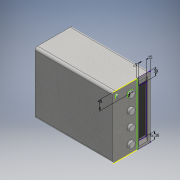
# Autodesk Inventor part: labortap1
Saved by Autodesk Inventor 2016 (Build 200138000, 138)
## iProperties
Created: 2017-12-27
Part Number: labortap1
Material: Generic
Document SubType Name: Modeling
Designer: Barna
Density: 1 g/cm^3
Appearance: Default
Author: Barna
Autodesk Inventor part; units mm, degrees
ref_plane "YZ Plane" through (0, 0, 0) normal (1, 0, 0) x (0, 1, 0)
ref_plane "XZ Plane" through (0, 0, 0) normal (0, 1, 0) x (-1, 0, 0)
ref_plane "XY Plane" through (0, 0, 0) normal (0, 0, 1) x (1, 0, 0)
sketch "Sketch1" plane through (0, 0, 0) normal (1, 0, 0) x (0, 1, 0)
  line L0 (0, 0) -> (155, 0)
  line L1 (155, 0) -> (155, -255)
  line L2 (155, -255) -> (0, -255)
  line L3 (0, -255) -> (0, 0)
  dimension "d1" = 255
  dimension "d2" = 155
  constraints: 8 end point, 2 parallel, 1 horizontal, 1 perpendicular
  measures "d1" distance of L0.end L1.end
  measures "d2" distance of L1.end L2.end
extrude "Extrusion1" add sketch "Sketch1" against normal blind 320
sketch "Sketch2" plane through (0, 0, 0) normal (1, 0, 0) x (0, 0, -1)
  line L0 (0, 0) -> (0, 155) projected
  line L1 (255, 155) -> (255, 0) projected
  line L2 (0, 155) -> (255, 155)
  line L3 (255, 155) -> (255, 99.4837)
  line L4 (255, 99.4837) -> (0, 99.4837)
  line L5 (0, 99.4837) -> (0, 155)
  line L6 (30, 140) -> (225, 140)
  line L7 (225, 140) -> (225, 104.4837)
  line L8 (225, 104.4837) -> (30, 104.4837)
  line L9 (30, 104.4837) -> (30, 140)
  dimension "d8" = 15
  dimension "d9" = 5
  dimension "d10" = 30
  dimension "d11" = 30
  constraints: 16 end point, 4 parallel, 2 horizontal, 2 perpendicular, 1 point on line
  measures "d8" distance between parallel lines of L6 L2
  measures "d9" distance between parallel lines of L4 L8
  measures "d10" distance between parallel lines of L0 L9
  measures "d11" distance between parallel lines of L1 L7
extrude "Extrusion2" add sketch "Sketch2" along normal blind 3 contours L0 L2 L1 L4 | L6 L7 L8 L9
fillet "Fillet1" radius 2 4 edges at (3, 155, -127.5) (3, 127.2418, 0) (3, 127.2418, -255) (3, 99.4837, -127.5)
extrude "Extrusion3" cut sketch "Sketch2" along normal blind 3 and the other way blind 5 contours L6 L7 L8 L9
chamfer "Chamfer2" distance 18 distance2 6 1 edges at (3, 122.2418, -30) measured on face at (3, 148.6667, -95)
chamfer "Chamfer3" distance 18 distance2 6 1 edges at (3, 122.2418, -225) measured on face at (3, 148.6667, -95)
sketch "Sketch3" plane through (0, 0, 0) normal (1, 0, 0) x (0, 0, -1)
  ellipse E0 centre (19.9684, 15.0609) end of major axis (26.6774, 15.0609) minor radius 4.7478
  circle A0 centre (40, 71.92) radius 12.5
  line L0 (0, 0) -> (0, 99.4837) projected
  dimension "d25" = 25
  dimension "d34" = 40
  constraints: 1 centre point, 2 other
  measures "d25" diameter of A0
  measures "d34" distance from line of A0.centre L0
extrude "Extrusion4" add sketch "Sketch3" along normal blind 8 contours E0
fillet "Fillet2" radius 2 1 edges at (8, 15.0609, -13.2594)
extrude "Extrusion5" add sketch "Sketch3" along normal blind 9 draft -4 contours A0
pattern_linear "Rectangular Pattern1" count 4 spacing 60 along (0, 0, -1) of "Extrusion5"
fillet "Fillet3" radius 10 6 edges at (-160, 0, 0) (2.4142, 154.4142, -0.5858) (-159.5, 155, 0) (-160, 0, -255) (2.4142, 154.4142, -254.4142) (-159.5, 155, -255)
equation "\"d11\" = d10"
body "Solid1"
